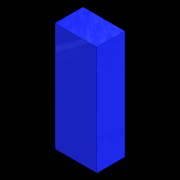
# Autodesk Inventor part: BatteryMockup
Saved by Autodesk Inventor 2022 (Build 260153000, 153)
## iProperties
Created: 2022-06-09
Part Number: BatteryMockup
Material: Generic
Document SubType Name: Modeling
Designer: tandu
Density: 1.6167 g/cm^3
Appearance: Blue - Wall Paint - Glossy
Mass: 55 g
Surface Area: 72.72 cm^2
Volume: 34.02 cm^3
Author: tandu
Autodesk Inventor part; units mm, degrees
ref_plane "YZ Plane" through (0, 0, 0) normal (1, 0, 0) x (0, 1, 0)
ref_plane "XZ Plane" through (0, 0, 0) normal (0, 1, 0) x (-1, 0, 0)
ref_plane "XY Plane" through (0, 0, 0) normal (0, 0, 1) x (1, 0, 0)
sketch "Sketch1" plane through (0, 0, 0) normal (0, 1, 0) x (-1, 0, 0)
  line L0 (-13.5, 9) -> (13.5, 9)
  line L1 (13.5, 9) -> (13.5, -9)
  line L2 (13.5, -9) -> (-13.5, -9)
  line L3 (-13.5, -9) -> (-13.5, 9)
  line L4 (-13.5, 9) -> (13.5, -9) construction
  line L5 (13.5, 9) -> (-13.5, -9) construction
  point P0 (0, 0)
  dimension "d0" = 27
  dimension "d1" = 18
  constraints: 12 end point, 2 midpoint, 2 parallel, 1 horizontal, 1 perpendicular
  measures "d0" distance of L1.end L2.end
  measures "d1" distance of L0.end L1.end
extrude "Extrusion1" add sketch "Sketch1" along normal blind 70
body "Solid1"
